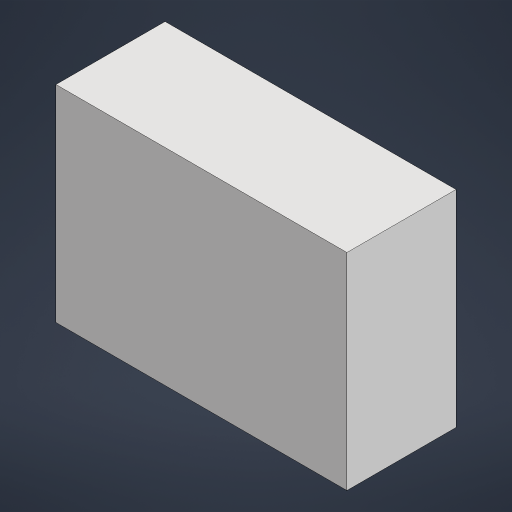
# Autodesk Inventor part: 34x18x48 - 3
Saved by Autodesk Inventor 2023.2 (Build 272271000, 271)
## iProperties
Created: 2022-12-08
Part Number: 34x18x48 - 3
Material: Generic
Document SubType Name: Modeling
Designer: awelt
Mass: 481386 g
Surface Area: 40103.1 cm^2
Volume: 481386 cm^3
Density: 1 g/cm^3
Appearance: Default
RuleStatus: InUse
BeforeDocSave0: file://C:\Users\awelt\Documents\Inventor\iLogic_Rules\BoundingStore
DocClose0: file://C:\Users\awelt\Documents\Inventor\iLogic_Rules\BoundingStore
Author: awelt
BoundingBL1: 18
BoundingBL2: 34
BoundingBL3: 48
BoundingCF: 17.0
Autodesk Inventor part; units mm, degrees
ref_plane "YZ Plane" through (0, 0, 0) normal (1, 0, 0) x (0, 1, 0)
ref_plane "XZ Plane" through (0, 0, 0) normal (0, 1, 0) x (-1, 0, 0)
ref_plane "XY Plane" through (0, 0, 0) normal (0, 0, 1) x (1, 0, 0)
sketch "Sketch2" plane through (0, 0, 0) normal (0, 1, 0) x (-1, 0, 0)
  line L0 (0, 0) -> (-1219.2, 0)
  line L1 (-1219.2, 0) -> (-1219.2, -457.2)
  line L2 (-1219.2, -457.2) -> (0, -457.2)
  line L3 (0, -457.2) -> (0, 0)
  dimension "d3" = 1219.2
  dimension "d4" = 457.2
  constraints: 8 end point, 2 parallel, 1 horizontal, 1 perpendicular
  measures "d3" distance of L2.end L1.end
  measures "d4" distance of L1.end L0.end
extrude "Extrusion1" add sketch "Sketch2" along normal blind 863.6
body "Solid1"
